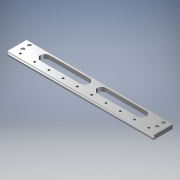
# Autodesk Inventor part: suporte_pincas
Saved by Autodesk Inventor 2018 (Build 220112000, 112)
## iProperties
Created: 2018-05-17
Part Number: suporte_pincas
Material: Alumínio 6061
Document SubType Name: Modeling
Designer: Usuario
Density: 2.7 g/cm^3
Appearance: Alumínio - Plano
Author: Usuario
Autodesk Inventor part; units mm, degrees
ref_plane "YZ Plane" through (0, 0, 0) normal (1, 0, 0) x (0, 1, 0)
ref_plane "XZ Plane" through (0, 0, 0) normal (0, 1, 0) x (-1, 0, 0)
ref_plane "XY Plane" through (0, 0, 0) normal (0, 0, 1) x (1, 0, 0)
sketch "Esboço1" plane through (0, 0, 0) normal (0, 0, 1) x (1, 0, 0)
  line L0 (-28, -30) -> (-28, 0) construction
  line L1 (0, -30) -> (-28, -30) construction
  line L2 (0, 0) -> (0, -30) construction
  line L3 (0, 0) -> (-28, 0) construction
  line L4 (286.8954, -30) -> (286.8954, 0) construction
  line L5 (314.8954, -30) -> (286.8954, -30) construction
  line L6 (314.8954, 0) -> (314.8954, -30) construction
  line L7 (314.8954, 0) -> (286.8954, 0) construction
  line L8 (-28, 0) -> (314.8954, 0)
  line L9 (314.8954, 0) -> (314.8954, -45)
  line L10 (314.8954, -45) -> (-28, -45)
  line L11 (-28, -45) -> (-28, 0)
  line L12 (-28, 0) -> (-28, -15) construction
  line L13 (143.4477, -15) -> (143.4477, 0) construction
  line L14 (0, -15) -> (40, -15) construction
  line L15 (143.4477, -15) -> (123.4477, -15) construction
  line L16 (143.4477, -15) -> (163.4477, -15) construction
  line L17 (40, -15) -> (123.4477, -15) construction
  line L18 (286.8954, -15) -> (256.8954, -15) construction
  line L19 (163.4477, -15) -> (256.8954, -15) construction
  line L20 (163.4477, -4) -> (256.8954, -4)
  line L21 (256.8954, -26) -> (163.4477, -26)
  arc A0 (163.4477, -4) -> (163.4477, -26) centre (163.4477, -15) ccw
  arc A1 (256.8954, -26) -> (256.8954, -4) centre (256.8954, -15) ccw
  line L22 (0, -15) -> (30, -15) construction
  line L23 (30, -15) -> (123.4477, -15) construction
  line L24 (30, -4) -> (123.4477, -4)
  line L25 (123.4477, -26) -> (30, -26)
  arc A2 (30, -4) -> (30, -26) centre (30, -15) ccw
  arc A3 (123.4477, -26) -> (123.4477, -4) centre (123.4477, -15) ccw
  line L26 (0, -37.5) -> (-28, -37.5) construction
  line L27 (0, -37.5) -> (286.8954, -37.5) construction
  line L28 (286.8954, -37.5) -> (314.8954, -37.5) construction
  circle A4 centre (0, -37.5) radius 2 construction
  circle A5 centre (31.87, -37.5) radius 2 construction
  circle A6 centre (63.74, -37.5) radius 2 construction
  circle A7 centre (95.61, -37.5) radius 2 construction
  circle A8 centre (127.48, -37.5) radius 2 construction
  circle A9 centre (159.35, -37.5) radius 2 construction
  circle A10 centre (191.22, -37.5) radius 2 construction
  circle A11 centre (223.09, -37.5) radius 2 construction
  circle A12 centre (254.96, -37.5) radius 2 construction
  circle A13 centre (286.83, -37.5) radius 2 construction
  circle A14 centre (-14, -7.5) radius 1.621 projected
  circle A15 centre (-14, -22.5) radius 1.621 projected
  circle A16 centre (300.8954, -7.5) radius 1.621 projected
  circle A17 centre (300.8954, -22.5) radius 1.621 projected
  point P0 (210.1715, -15)
  point P1 (76.7238, -15)
  dimension "d0" = 45
  dimension "d1" = 15
  dimension "d3" = 20
  dimension "d4" = 20
  dimension "d7" = 30
  dimension "d8" = 93.4477
  dimension "d9" = 30
  dimension "d12" = 286.8954
  dimension "d15" = 4
  dimension "d18" = 31.87
  constraints: 48 end point, 14 centre point, 8 point on circle, 8 tangent, 5 midpoint, 5 point on line, 4 parallel, 3 horizontal, 2 collinear, 2 perpendicular, 1 coincident, 18 other
  measures "d0" distance of L8.end L9.end
  measures "d1" distance of L0.end L12.end
  measures "d3" distance of L13.start L15.end
  measures "d4" distance of L13.start L16.end
  measures "d7" distance of L18.start L18.end
  measures "d8" distance of L21.start L21.end
  measures "d9" distance of L14.start L22.end
  measures "d12" distance of L26.start L27.end
  measures "d15" diameter of A4
  measures "d18" distance of A4.centre A5.centre
extrude "Extrusão1" add sketch "Esboço1" along normal blind 9.55 contours L8 L9 L10 L11 | A14 | A15 | A16 | A17
sketch "Esboço2" plane through (0, 0, 9.55) normal (0, 0, 1) x (1, 0, 0)
  line L0 (-28, -45) -> (-28, -35) construction
  line L1 (-28, -35) -> (314.8954, -35) construction
  line L2 (-7.5636, -30) -> (-7.5636, -2) construction
  line L3 (294.3318, -30) -> (294.3318, -2) construction
  circle A0 centre (-7.5636, -35) radius 2 construction
  circle A1 centre (25.9364, -35) radius 2 construction
  circle A2 centre (59.4364, -35) radius 2 construction
  circle A3 centre (92.9364, -35) radius 2 construction
  circle A4 centre (126.4364, -35) radius 2 construction
  circle A5 centre (159.9364, -35) radius 2 construction
  circle A6 centre (193.4364, -35) radius 2 construction
  circle A7 centre (226.9364, -35) radius 2 construction
  circle A8 centre (260.4364, -35) radius 2 construction
  circle A9 centre (293.9364, -35) radius 2 construction
  point P0 (0, 0)
  dimension "d25" = 10
  dimension "d26" = 4
  dimension "d29" = 33.5
  constraints: 10 centre point, 8 end point, 2 vertical, 1 horizontal, 1 perpendicular, 1 point on line, 22 other
  measures "d25" distance of L0.start L0.end
  measures "d26" diameter of A0
  measures "d29" distance of A0.centre A1.centre
sketch "Esboço3" plane through (-28, -45, 0) normal (-1, 0, 0) x (0, 0, 1)
  line L0 (9.55, 0) -> (14.9508, 0) construction
  line L1 (9.55, 45) -> (9.55, 0) projected
  line L2 (3.84, -43.6324) -> (3.84, -46.1668) construction
  line L3 (0, 0) -> (9.55, 0) projected
  line L4 (3.84, 0) -> (7.0867, 0)
  line L5 (3.84, 0) -> (3.84, 3)
  line L6 (3.84, 3) -> (9.55, 0)
  point P0 (0, 45)
  point P1 (4.775, 0)
  dimension "d58" = 3
  constraints: 8 end point, 2 horizontal, 1 point on line, 1 vertical
  measures "d58" distance of L4.start L5.end
extrude "Extrusão2" cut sketch "Esboço3" against normal up to next
sketch "Esboço4" plane through (0, 0, 9.55) normal (0, 0, 1) x (1, 0, 0)
  circle A0 centre (-14, -7.5) radius 1.621 construction
  circle A1 centre (-14, -22.5) radius 1.621 construction
  circle A2 centre (300.8954, -7.5) radius 1.621 construction
  circle A3 centre (300.8954, -22.5) radius 1.621 construction
  point P0 (0, 0)
hole "Furo2" at (-14, -7.5, 9.55) at (-14, -22.5, 9.55) at (300.8954, -7.5, 9.55) at (300.8954, -22.5, 9.55) direction (0, 0, -1) diameter 4 end through all counterbore diameter 8 counterbore depth 4.3
hole "Furo3" at (-7.5636, -35, 9.55) at (25.9364, -35, 9.55) at (59.4364, -35, 9.55) at (92.9364, -35, 9.55) at (126.4364, -35, 9.55) at (159.9364, -35, 9.55) at (193.4364, -35, 9.55) at (226.9364, -35, 9.55) at (260.4364, -35, 9.55) at (293.9364, -35, 9.55) direction (0, 0, -1) diameter 4.917 end through all thread size "M6x1" class "6H" standard "ANSI Metric M Profile"
